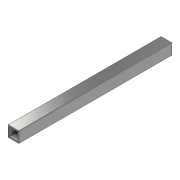
# Autodesk Inventor part: 16x16x2 voor noodstop
Saved by Autodesk Inventor 2020.3 (Build 243373000, 373)
## iProperties
Created: 2020-12-02
Part Number: 16x16x2 voor noodstop
Material: Stainless Steel
Document SubType Name: Modeling
Designer: Svend
Density: 8 g/cm^3
Appearance: Semi-Polished
Author: Svend
Autodesk Inventor part; units mm, degrees
ref_plane "YZ Plane" through (0, 0, 0) normal (1, 0, 0) x (0, 1, 0)
ref_plane "XZ Plane" through (0, 0, 0) normal (0, 1, 0) x (-1, 0, 0)
ref_plane "XY Plane" through (0, 0, 0) normal (0, 0, 1) x (1, 0, 0)
sketch "Sketch1" plane through (0, 0, 0) normal (0, 0, 1) x (1, 0, 0)
  line L0 (-8, 8) -> (8, 8)
  line L1 (8, 8) -> (8, -8)
  line L2 (8, -8) -> (-8, -8)
  line L3 (-8, -8) -> (-8, 8)
  line L4 (-8, 8) -> (8, -8) construction
  line L5 (8, 8) -> (-8, -8) construction
  line L6 (6, 6) -> (-6, 6)
  line L7 (-6, 6) -> (-6, -6)
  line L8 (-6, -6) -> (6, -6)
  line L9 (6, -6) -> (6, 6)
  point P0 (0, 0)
  dimension "d0" = 16
  dimension "d1" = 16
  dimension "d2" = 2
  constraints: 20 end point, 4 parallel, 2 midpoint, 2 perpendicular, 1 horizontal, 3 other
  measures "d0" distance of L1.end L2.end
  measures "d1" distance of L0.end L1.end
  measures "d2" distance between parallel lines of L0 L6
extrude "Extrusion1" add sketch "Sketch1" along normal blind 220
fillet "Fillet1" radius 0.5 24 edges at (-6, 0, 0) (6, 0, 0) (0, -6, 0) (0, 6, 0) (0, -8, 0) (0, 8, 0) (-8, 8, 110) (-8, -8, 110) (-6, 0, 220) (-6, -6, 110) (-6, 6, 110) (0, -6, 220) (0, 6, 220) (0, -8, 220) (0, 8, 220) (6, 0, 220) (6, -6, 110) (6, 6, 110) (8, 0, 220) (8, -8, 110) (8, 8, 110) (8, 0, 0) (-8, 0, 0) (-8, 0, 220)
body "Solid1"
